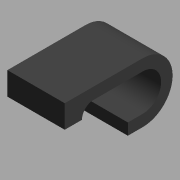
# Autodesk Inventor part: lid_holder
Saved by Autodesk Inventor 2019 (Build 230136000, 136)
## iProperties
Part Number: lid_holder
Material: Generic
Document SubType Name: Modeling
Designer: Javi
Appearance: Default
Author: Javi
Autodesk Inventor part; units mm, degrees
ref_plane "YZ Plane" through (0, 0, 0) normal (1, 0, 0) x (0, 1, 0)
ref_plane "XZ Plane" through (0, 0, 0) normal (0, 1, 0) x (-1, 0, 0)
ref_plane "XY Plane" through (0, 0, 0) normal (0, 0, 1) x (1, 0, 0)
sketch "Sketch1" plane through (0, 0, 0) normal (1, 0, 0) x (0, 1, 0)
  line L0 (10, 0) -> (10, -13)
  line L1 (0, 0) -> (0, -13)
  line L2 (52, -13) -> (52, 55)
  line L3 (52, 55) -> (32, 55)
  line L4 (52, 55) -> (72, 55) construction
  line L5 (32, 55) -> (32, 40)
  line L6 (32, 55) -> (47, 55) construction
  line L7 (32, 40) -> (32, 40)
  line L8 (42, 30) -> (42, -13)
  arc A0 (42, 30) -> (32, 40) centre (32, 30) ccw
  arc A1 (10, -13) -> (42, -13) centre (26, -13) ccw
  arc A2 (0, -13) -> (52, -13) centre (26, -13) ccw
  line L9 (0, 0) -> (10, 0)
  dimension "d2" = 13
  dimension "d7" = 13
  dimension "d12" = 68
  dimension "d14" = 20
  dimension "d16" = 15
  dimension "d19" = 10
  dimension "d20" = 16
  dimension "d21" = 26
  dimension "d22" = 10
  constraints: 20 end point, 6 point on circle, 6 tangent, 5 vertical, 4 horizontal, 3 centre point, 2 equal length, 1 perpendicular
  measures "d2" distance of L0.start L0.end
  measures "d7" distance of L1.start L1.end
  measures "d12" distance of L2.start L2.end
  measures "d14" distance of L2.end L3.end
  measures "d16" distance of L3.end L5.end
  measures "d19" radius of A0
  measures "d20" radius of A1
  measures "d21" radius of A2
  measures "d22" distance of L1.start L0.start
extrude "Extrusion1" add sketch "Sketch1" along normal blind 50
sketch "Sketch2" plane through (0, 32, 40) normal (0, -1, 0) x (1, 0, 0)
  circle A0 centre (10, 7.5) radius 2
  line L0 (0, 15) -> (0, 0) projected
  line L1 (0, 15) -> (50, 15) projected
  circle A1 centre (40, 7.5) radius 2
  point P0 (0, -40)
  dimension "d25" = 4
  dimension "d26" = 10
  dimension "d27" = 7.5
  dimension "d30" = 30
  constraints: 2 centre point, 1 horizontal, 2 other
  measures "d25" diameter of A0
  measures "d26" distance from line of L0 A0.centre
  measures "d27" distance from line of L1 A0.centre
  measures "d30" distance of A0.centre A1.centre
extrude "Extrusion2" cut sketch "Sketch2" against normal blind 15
body "Solid1"
